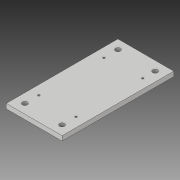
# Autodesk Inventor part: GalvoBoardPlate_V2
Saved by Autodesk Inventor 2019 (Build 230136000, 136)
## iProperties
Created: 2021-08-16
Part Number: GalvoBoardPlate_V2
Material: Generic
Document SubType Name: Modeling
Designer: devon
Density: 1 g/cm^3
Appearance: Default
Author: devon
Autodesk Inventor part; units mm, degrees
ref_plane "YZ Plane" through (0, 0, 0) normal (1, 0, 0) x (0, 1, 0)
ref_plane "XZ Plane" through (0, 0, 0) normal (0, 1, 0) x (-1, 0, 0)
ref_plane "XY Plane" through (0, 0, 0) normal (0, 0, 1) x (1, 0, 0)
sketch "Sketch1" plane through (0, 0, 0) normal (0, 1, 0) x (-1, 0, 0)
  line L0 (38.1, 76.2) -> (-38.1, 76.2)
  line L1 (-38.1, 76.2) -> (-38.1, -76.2)
  line L2 (-38.1, -76.2) -> (38.1, -76.2)
  line L3 (38.1, -76.2) -> (38.1, 76.2)
  line L4 (38.1, 76.2) -> (-38.1, -76.2) construction
  line L5 (-38.1, 76.2) -> (38.1, -76.2) construction
  point P0 (0, 0)
  dimension "d0" = 76.2
  dimension "d1" = 152.4
  constraints: 12 end point, 2 midpoint, 2 parallel, 1 horizontal, 1 perpendicular
  measures "d0" distance of L1.end L2.end
  measures "d1" distance of L0.end L1.end
extrude "Extrusion1" add sketch "Sketch1" along normal blind 6.35
sketch "Sketch2" plane through (0, 6.35, 0) normal (0, 1, 0) x (1, 0, 0)
  line L0 (38.1, 76.2) -> (-38.1, 76.2) projected
  line L1 (-38.1, 76.2) -> (-38.1, -76.2) projected
  line L2 (38.1, -76.2) -> (38.1, 76.2) projected
  line L3 (-38.1, -76.2) -> (38.1, -76.2) projected
  point P0 (0, 0)
  point P1 (-25.4, 63.5)
  point P2 (25.4, 63.5)
  point P3 (25.4, -63.5)
  point P4 (-25.4, -63.5)
  dimension "d11" = 12.7
  dimension "d12" = 12.7
  dimension "d13" = 12.7
  dimension "d14" = 12.7
  dimension "d15" = 12.7
  dimension "d16" = 12.7
  dimension "d17" = 12.7
  dimension "d18" = 12.7
  measures "d11" distance from line of L0 point (-25.4, 63.5)
  measures "d12" distance from line of L1 point (-25.4, 63.5)
  measures "d13" distance from line of L0 point (25.4, 63.5)
  measures "d14" distance from line of L2 point (25.4, 63.5)
  measures "d15" distance from line of L1 point (-25.4, -63.5)
  measures "d16" distance from line of L3 point (-25.4, -63.5)
  measures "d17" distance from line of L3 point (25.4, -63.5)
  measures "d18" distance from line of L2 point (25.4, -63.5)
hole "Hole1" at (-25.4, 6.35, -63.5) at (25.4, 6.35, -63.5) at (25.4, 6.35, 63.5) at (-25.4, 6.35, 63.5) direction (0, -1, 0) diameter 6.7564 depth 10.8 tip angle 118 clearance for "Socket Head Cap Screw" size "1/4" standard "Ansi Unified Screw Threads"
sketch "Sketch3" plane through (0, 6.35, 0) normal (0, 1, 0) x (1, 0, 0)
  line L0 (-38.1, -76.2) -> (38.1, -76.2) projected
  line L1 (-38.1, 76.2) -> (-38.1, -76.2) projected
  line L2 (38.1, -76.2) -> (38.1, 76.2) projected
  line L3 (38.1, 76.2) -> (-38.1, 76.2) projected
  point P0 (0, 0)
  point P1 (-25.4, 44.45)
  point P2 (-25.4, -44.45)
  point P3 (25.4, -44.45)
  point P4 (25.4, 46.482)
  dimension "d26" = 31.75
  dimension "d27" = 12.7
  dimension "d28" = 31.75
  dimension "d29" = 12.7
  dimension "d30" = 12.7
  dimension "d32" = 31.75
  dimension "d33" = 12.7
  dimension "d34" = 90.932
  measures "d26" distance from line of L0 point (-25.4, -44.45)
  measures "d27" distance from line of L1 point (-25.4, -44.45)
  measures "d28" distance from line of L0 point (25.4, -44.45)
  measures "d29" distance from line of L2 point (25.4, -44.45)
  measures "d30" distance from line of L2 point (25.4, 46.482)
  measures "d32" distance from line of L3 point (-25.4, 44.45)
  measures "d33" distance from line of L1 point (-25.4, 44.45)
  measures "d34" distance of point (25.4, -44.45) point (25.4, 46.482)
hole "Hole2" at (-25.4, 6.35, -44.45) at (-25.4, 6.35, 44.45) at (25.4, 6.35, 44.45) at (25.4, 6.35, -46.482) direction (0, -1, 0) diameter 2.6416 depth 10.9728 tip angle 118 thread size "6-32 UNC" class "2B" standard "ANSI Unified Screw Threads"
body "Solid1"
